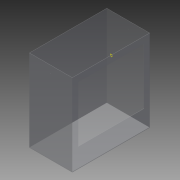
# Autodesk Inventor part: box_middlegoalLOW
Saved by Autodesk Inventor 2013 (Build 170138000, 138)
## iProperties
Created: 2012-12-31
Part Number: box_middlegoalLOW
Material: Polycarbonate, Clear
Document SubType Name: Modeling
Designer: Phillip
Density: 1 g/cm^3
Author: Phillip
Autodesk Inventor part; units mm, degrees
ref_plane "YZ Plane" through (0, 0, 0) normal (1, 0, 0) x (0, 1, 0)
ref_plane "XZ Plane" through (0, 0, 0) normal (0, 1, 0) x (-1, 0, 0)
ref_plane "XY Plane" through (0, 0, 0) normal (0, 0, 1) x (1, 0, 0)
sketch "Sketch1" plane through (0, 0, 0) normal (0, 0, 1) x (1, 0, 0)
  line L0 (-457.2, -254) -> (457.2, -254)
  line L1 (457.2, -254) -> (457.2, 254)
  line L2 (457.2, 254) -> (-457.2, 254)
  line L3 (-457.2, 254) -> (-457.2, -254)
  line L4 (-457.2, -254) -> (457.2, 254) construction
  line L5 (457.2, -254) -> (-457.2, 254) construction
  point P0 (0, 0)
  dimension "d0" = 914.4
  dimension "d1" = 508
  constraints: 12 end point, 2 midpoint, 2 parallel, 1 horizontal, 1 perpendicular
  measures "d0" distance of L2.end L1.end
  measures "d1" distance of L1.end L0.end
extrude "Extrusion1" add sketch "Sketch1" against normal blind 965.2
shell "Shell1" thickness 3.175 removed faces 1 at (-152.4, 84.6667, 0)
sketch "Sketch2" plane through (-457.2, -254, 0) normal (0, -1, 0) x (1, 0, 0)
  line L0 (0, 0) -> (0, -965.2) projected
  line L1 (914.4, -965.2) -> (0, -965.2) projected
  line L2 (69.85, -76.2) -> (844.55, -76.2)
  line L3 (844.55, -76.2) -> (844.55, -736.6)
  line L4 (844.55, -736.6) -> (69.85, -736.6)
  line L5 (69.85, -736.6) -> (69.85, -76.2)
  point P0 (457.2, 0)
  dimension "d5" = 69.85
  dimension "d6" = 774.7
  dimension "d7" = 660.4
  dimension "d8" = 228.6
  constraints: 8 end point, 2 parallel, 1 horizontal, 1 perpendicular
  measures "d5" distance between parallel lines of L5 L0
  measures "d6" distance of L2.start L2.end
  measures "d7" distance of L4.end L2.start
  measures "d8" distance between parallel lines of L1 L4
extrude "Extrusion2" cut sketch "Sketch2" against normal up to next
sketch "Sketch3" plane through (-457.2, -254, 0) normal (-1, 0, 0) x (0, 0, 1)
  point P0 (0, 254)
  point P1 (-83.6587, 254)
hole "Hole1" at (-457.2, 0, -83.6587) direction (1, 0, 0) diameter 6.35 end through all
ref_plane "Work Plane1" through (0, -254, 0) normal (1, 0, 0) x (0, 1, 0)
body "Solid1"
